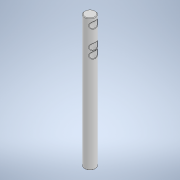
# Autodesk Inventor part: 80. Шток первой и второй передач
Saved by Autodesk Inventor 2021 (Build 250183000, 183)
## iProperties
Created: 2021-03-18
Part Number: 80. Шток первой и второй передач
Material: Типовые
Document SubType Name: Modeling
Designer: Данил
Density: 1 g/cm^3
Appearance: По умолчанию
Author: Данил
Autodesk Inventor part; units mm, degrees
ref_plane "YZ Plane" through (0, 0, 0) normal (1, 0, 0) x (0, 1, 0)
ref_plane "XZ Plane" through (0, 0, 0) normal (0, 1, 0) x (-1, 0, 0)
ref_plane "XY Plane" through (0, 0, 0) normal (0, 0, 1) x (1, 0, 0)
sketch "Эскиз1" plane through (0, 0, 0) normal (0, 0, 1) x (1, 0, 0)
  line L0 (0, 91.5) -> (0, -91.5)
  line L1 (0, -91.5) -> (6.75, -91.5)
  line L2 (7.5, -90.75) -> (7.5, 90.75)
  line L3 (6.75, 91.5) -> (0, 91.5)
  line L4 (7.5, -90.75) -> (6.75, -91.5)
  line L5 (7.5, 90.75) -> (6.75, 91.5)
  point P0 (0, 0)
  point P1 (0, 0)
  point P2 (7.5, -91.5)
  point P3 (7.5, 91.5)
  dimension "d0" = 183
  dimension "d1" = 15
  dimension "d2" = 0.75
  dimension "d3" = 45
  dimension "d4" = 0.75
  dimension "d5" = 45
  constraints: 12 end point, 4 point on line, 2 perpendicular, 1 coincident, 1 horizontal, 1 midpoint, 1 vertical
  measures "d0" distance of L0.start L0.end
  measures "d1" diameter of L2 L0
  measures "d2" distance of L2.start point (7.5, -91.5)
  measures "d3" angle of L2 L4
  measures "d4" distance of L2.end point (7.5, 91.5)
  measures "d5" angle of L2 L5
revolve "Вращение1" add sketch "Эскиз1" angle 360 about axis through (0, 91.5, 0) along (0, -1, 0)
sketch "Эскиз2" plane through (0, 0, 0) normal (0, 0, 1) x (1, 0, 0)
  arc A0 (7.5, 86.8128) -> (7.5, 78.1872) centre (9.1, 82.5) ccw
  line L0 (7.5, 90.75) -> (7.5, -90.75) projected
  line L1 (-7.5, 90.75) -> (-7.5, -90.75) projected
  line L2 (-6.75, 91.5) -> (6.75, 91.5) projected
  point P0 (0, 0)
  point P1 (4.5, 82.5)
  dimension "d7" = 12
  dimension "d8" = 4.6
  dimension "d9" = 9
  constraints: 3 point on circle, 2 point on line, 1 centre point, 1 horizontal alignment
  measures "d7" distance from line of L1 point (4.5, 82.5)
  measures "d8" radius of A0
  measures "d9" distance from line of L2 point (4.5, 82.5)
extrude "Выдавливание1" cut sketch "Эскиз2" against normal through all both and the other way through all
pattern_linear "Прямоуг.массив1" count 2 spacing 26 along (0, -1, 0) of "Выдавливание1"
pattern_linear "Прямоуг.массив2" count 2 spacing 10 along (0, -1, 0) of "Прямоуг.массив1"
fillet "Сопряжение1" radius 0.8 6 edges at (4.5, 46.4957, -6) (4.5, 46.4957, 6) (4.5, 56.4957, -6) (4.5, 56.4957, 6) (4.5, 82.4957, 6) (4.5, 82.4957, -6)
equation "\"d4\" = d2"
equation "\"d5\" = d3"
